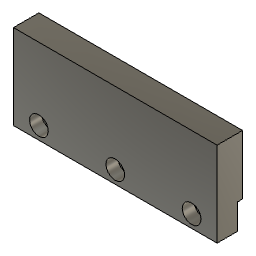
연습예제_2 (Autodesk Fusion 360 design; units mm, degrees)
Autodesk Fusion 360 part; units mm, degrees
sketch "Sketch1" plane through (0, 0, 0) normal (0, 1, 0) x (1, 0, 0)
  line L0 (-60, 0) -> (60, 0)
  line L1 (60, 0) -> (60, -50)
  line L2 (60, -50) -> (-60, -50)
  line L3 (-60, -50) -> (-60, 0)
  line L4 (-60, -15) -> (60, -15)
  dimension "d1" = 120
  dimension "d2" = 50
  dimension "d3" = 15
  constraint horizontal L0
  constraint vertical L1
  constraint horizontal L2
  constraint vertical L3
  constraint midpoint origin L0
  constraint coincident L3 L4.start
  constraint coincident L1 L4.end
  constraint perpendicular L1 L4
  measures "d1" distance of L0.start L0.end
  measures "d2" distance of L0.end L1.end
  measures "d3" distance of L0 L4
extrude "Extrude1" add sketch "Sketch1" along normal blind 15 contours L1 L2 L3 L4
extrude "Extrude2" add sketch "Sketch1" along normal blind 12 contours L0 L1 L3 L4
sketch "Sketch4" plane through (0, 0, 0) normal (0, -1, 0) x (1, 0, 0)
  line L0 (-60, 0) -> (-60, 15)
  line L1 (-60, 7.5) -> (-45, 7.5)
  line L2 (-60, 0) -> (60, 0)
  line L3 (-45, 7.5) -> (0, 7.5)
  line L4 (0, 7.5) -> (45, 7.5)
  line L5 (60, 15) -> (60, 0)
  line L6 (45, 7.5) -> (60, 7.5)
  dimension "d9" = 15
  dimension "d10" = 7.5
  dimension "d11" = 45
  dimension "d12" = 45
  constraint coincident L0 L1.start
  constraint perpendicular L0 L1
  constraint perpendicular L0 L3
  constraint parallel L3 L4
  constraint midpoint L5 L6.end
  measures "d9" distance of L1.start L1.end
  measures "d10" distance of L1 L2
  measures "d11" distance of L1.end L3.end
  measures "d12" distance of L3.end L4.end
hole "Hole1" at (-45, 0, 7.5) at (45, 0, 7.5) at (0, 0, 7.5) direction (0, 1, 0) diameter 6.036 depth 11 tip angle 118 counterbore diameter 11 counterbore depth 7
thread "Thread1" "ISO Metric profile 7.0 M7x1 6H" thread offset 0 thread depth 9.9
